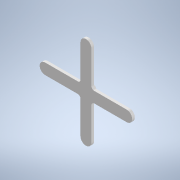
# Autodesk Inventor part: Adapter_Drehteller
Saved by Autodesk Inventor 2021 (Build 250183000, 183)
## iProperties
Created: 2022-06-25
Part Number: Adapter_Drehteller
Material: Generisch
Document SubType Name: Modeling
Designer: adria
Density: 1 g/cm^3
Appearance: Vorgabe
Mass: 31.7515 g
Surface Area: 159.363 cm^2
Volume: 31.7515 cm^3
Author: adria
Autodesk Inventor part; units mm, degrees
ref_plane "YZ Plane" through (0, 0, 0) normal (1, 0, 0) x (0, 1, 0)
ref_plane "XZ Plane" through (0, 0, 0) normal (0, 1, 0) x (-1, 0, 0)
ref_plane "XY Plane" through (0, 0, 0) normal (0, 0, 1) x (1, 0, 0)
sketch "Skizze1" plane through (0, 0, 0) normal (0, 0, 1) x (1, 0, 0)
  circle A0 centre (0, 0) radius 4
  dimension "d0" = 8
  constraints: 1 centre point, 1 coincident
  measures "d0" diameter of A0
extrude "Extrusion1" add sketch "Skizze1" along normal blind 10
sketch "Skizze2" plane through (0, 0, 10) normal (0, 0, 1) x (1, 0, 0)
  circle A0 centre (0, 0) radius 4 projected
  line L0 (-75, 10) -> (-15, 10)
  arc A1 (-15, 10) -> (-10, 15) centre (-15, 15) ccw
  arc A2 (10, 75) -> (-10, 75) centre (0, 75) ccw
  line L1 (0, -121.8995) -> (0, 121.8995) projected
  line L2 (-10, 75) -> (-10, 15)
  line L3 (-121.8995, 0) -> (121.8995, 0) projected
  arc A3 (-75, 10) -> (-85, 0) centre (-75, 0) ccw
  circle A4 centre (0, 75) radius 3.05
  arc A5 (-10, -75) -> (0, -85) centre (0, -75) ccw
  line L4 (-10, -75) -> (-10, -15)
  arc A6 (-10, -15) -> (-15, -10) centre (-15, -15) ccw
  line L5 (-75, -10) -> (-15, -10)
  arc A7 (-75, 10) -> (-75, -10) centre (-75, 0) ccw
  circle A8 centre (-75, 0) radius 3.05
  arc A9 (75, -10) -> (85, 0) centre (75, 0) ccw
  line L6 (75, -10) -> (15, -10)
  arc A10 (15, -10) -> (10, -15) centre (15, -15) ccw
  line L7 (10, -75) -> (10, -15)
  arc A11 (-10, -75) -> (10, -75) centre (0, -75) ccw
  circle A12 centre (0, -75) radius 3.05
  arc A13 (10, 75) -> (0, 85) centre (0, 75) ccw
  line L8 (10, 75) -> (10, 15)
  arc A14 (10, 15) -> (15, 10) centre (15, 15) ccw
  line L9 (75, 10) -> (15, 10)
  arc A15 (75, -10) -> (75, 10) centre (75, 0) ccw
  circle A16 centre (75, 0) radius 3.05
  point P0 (-85, 0)
  point P1 (0, -85)
  point P2 (85, 0)
  point P3 (10, 75)
  dimension "d3" = 10
  dimension "d4" = 5
  dimension "d5" = 10
  dimension "d6" = 75
  dimension "d7" = 75
  dimension "d8" = 6.1
  dimension "d11" = 360
  constraints: 28 point on circle, 16 centre point, 16 end point, 7 coincident, 4 point on line, 4 tangent, 1 horizontal, 1 vertical, 71 other
  measures "d3" distance between parallel lines of L1 L2
  measures "d4" radius of A1
  measures "d5" distance between parallel lines of L3 L0
  measures "d6" distance of A0.centre A2.centre
  measures "d7" distance of A3.centre A0.centre
  measures "d8" diameter of A4
extrude "Extrusion2" add sketch "Skizze2" along normal blind 5 contours L3 L1 A0 | L3 A16 A9 L6 A10 L7 A11 L1 A12 A0 | A0 L1 L3 | A0 L1 A4 A2 L8 A14 L9 A15 L3 A16 | L1 L3 A0 | A0 L3 A8 A3 L0 A1 L2 A2 L1 A4 | L1 A12 A5 L4 A6 L5 A7 L3 A8 A0 | A0 L3 L1
sketch "Skizze3" plane through (0, 0, 15) normal (0, 0, 1) x (1, 0, 0)
  circle A0 centre (0, -75) radius 3.05 projected
  circle A1 centre (75, 0) radius 3.05 projected
  circle A2 centre (0, 75) radius 3.05 projected
  circle A3 centre (-75, 0) radius 3.05 projected
  point P0 (0, 0)
extrude "Extrusion3" add sketch "Skizze3" against normal up to surface (5 mm away)
